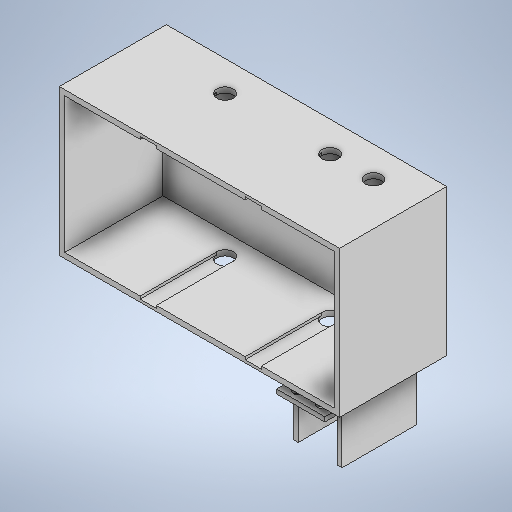
# Autodesk Inventor part: ClawHousing
Saved by Autodesk Inventor 2025.1 (Build 291241000, 241)
## iProperties
Created: 2024-12-07
Part Number: ClawHousing
Material: Generic
Document SubType Name: Modeling
Designer: ishaa
Density: 1 g/cm^3
Appearance: Default
Author: ishaa
Autodesk Inventor part; units mm, degrees
ref_plane "YZ Plane" through (0, 0, 0) normal (1, 0, 0) x (0, 1, 0)
ref_plane "XZ Plane" through (0, 0, 0) normal (0, 1, 0) x (-1, 0, 0)
ref_plane "XY Plane" through (0, 0, 0) normal (0, 0, 1) x (1, 0, 0)
sketch "Sketch1" plane through (0, 0, 0) normal (0, 0, 1) x (1, 0, 0)
  line L0 (78.5, 41) -> (-78.5, 41)
  line L1 (-78.5, 41) -> (-78.5, -41)
  line L2 (-78.5, -41) -> (78.5, -41)
  line L3 (78.5, -41) -> (78.5, 41)
  line L4 (78.5, 41) -> (-78.5, -41) construction
  line L5 (-78.5, 41) -> (78.5, -41) construction
  point P0 (0, 0)
  dimension "d0" = 157
  dimension "d1" = 82
  constraints: 12 end point, 2 midpoint, 2 parallel, 1 horizontal, 1 perpendicular
  measures "d0" distance of L2.end L1.end
  measures "d1" distance of L1.end L0.end
extrude "Extrusion1" add sketch "Sketch1" along normal blind 60
sketch "Sketch2" plane through (0, 0, 60) normal (0, 0, 1) x (1, 0, 0)
  line L0 (-78.5, 41) -> (-78.5, -41) projected
  line L1 (-78.5, -41) -> (78.5, -41) projected
  line L2 (78.5, -41) -> (78.5, 41) projected
  line L3 (78.5, 41) -> (-78.5, 41) projected
  line L4 (75.5, 38) -> (75.5, -38)
  line L5 (75.5, -38) -> (-75.5, -38)
  line L6 (-75.5, -38) -> (-75.5, 38)
  line L7 (-75.5, 38) -> (75.5, 38)
  point P0 (0, 0)
  dimension "d4" = 3
  constraints: 8 end point, 3 other
  measures "d4" distance between parallel lines of L2 L4
extrude "Extrusion2" cut sketch "Sketch2" against normal blind 55 contours L4 L5 L6 L7
sketch "Sketch3" plane through (-78.5, -41, 0) normal (0, -1, 0) x (1, 0, 0)
  circle A0 centre (133, 17) radius 4.55 construction
  line L0 (0, 0) -> (157, 0) construction
  line L1 (133, 0) -> (133, 85.8256) construction
  line L2 (157, 0) -> (157, 60) construction
  circle A1 centre (108.668, 17) radius 4.55
  line L3 (154, 60) -> (3, 60) construction
  line L4 (0, 0) -> (0, 60) construction
  circle A2 centre (49.832, 17) radius 4.55
  line L5 (157, 17) -> (0, 17) construction
  circle A3 centre (133, 17) radius 6.75
  point P0 (78.5, 0)
  point P1 (128.45, 17)
  point P2 (113.218, 17)
  dimension "d7" = 9.1
  dimension "d11" = 9.1
  dimension "d15" = 9.1
  dimension "d19" = 24.332
  constraints: 8 point on line, 4 end point, 2 centre point, 2 coincident, 2 horizontal alignment, 1 perpendicular, 1 vertical, 5 other
  measures "d15" diameter of A2
  measures "d19" distance of point (133, 17) point (108.668, 17)
extrude "Extrusion3" cut sketch "Sketch3" against normal blind 60
sketch "Sketch4" plane through (-78.5, 41, 0) normal (0, 1, 0) x (1, 0, 0)
  circle A0 centre (49.832, -17) radius 4.55
  line L0 (157, -60) -> (0, -60) construction
  line L1 (157, 0) -> (157, -60) construction
  line L2 (157, 0) -> (0, 0) construction
  line L3 (0, 0) -> (0, -60) construction
  circle A1 centre (133, -17) radius 6.75 construction
  circle A2 centre (133, -17) radius 4.55
  circle A3 centre (108.668, -17) radius 4.55
  dimension "d70" = 9.1
  dimension "d71" = 9.1
  dimension "d72" = 24.332
  constraints: 3 centre point, 2 coincident
  measures "d70" diameter of A2
  measures "d71" diameter of A3
  measures "d72" distance of A1.centre A3.centre
extrude "Extrusion4" cut sketch "Sketch4" against normal blind 55
sketch "Sketch5" plane through (0, 0, 0) normal (0, 0, -1) x (-1, 0, 0)
  line L0 (8, 13.8564) -> (16, 0) construction
  line L1 (16, 0) -> (8, -13.8564) construction
  line L2 (8, -13.8564) -> (-8, -13.8564) construction
  line L3 (-8, -13.8564) -> (-16, 0) construction
  line L4 (-16, 0) -> (-8, 13.8564) construction
  line L5 (-8, 13.8564) -> (8, 13.8564) construction
  circle A0 centre (-8, 13.8564) radius 1.675
  circle A1 centre (-16, 0) radius 1.675
  circle A2 centre (-8, -13.8564) radius 1.675
  circle A3 centre (8, -13.8564) radius 1.675
  circle A4 centre (16, 0) radius 1.675
  circle A5 centre (8, 13.8564) radius 1.675
  point P0 (0, 0)
  point P1 (0, 0)
  dimension "d31" = 32
  dimension "d32" = 3.35
  dimension "d35" = 360
  constraints: 12 end point, 6 centre point, 2 coincident, 26 other
  measures "d31" distance of L0.end L3.end
  measures "d32" diameter of A0
extrude "Extrusion5" cut sketch "Sketch5" against normal blind 55
chamfer "Chamfer1" distance 1 angle 45 6 edges at (-6.325, -13.8564, 0) (9.675, -13.8564, 0) (17.675, 0, 0) (9.675, 13.8564, 0) (-6.325, 13.8564, 0) (-14.325, 0, 0)
sketch "Sketch6" plane through (0, 0, 0) normal (0, 0, -1) x (-1, 0, 0)
  line L0 (0, -4.344) -> (-3.762, -2.172)
  line L1 (-3.762, -2.172) -> (-3.762, 2.172)
  line L2 (-3.762, 2.172) -> (0, 4.344)
  line L3 (0, 4.344) -> (3.762, 2.172)
  line L4 (3.762, 2.172) -> (3.762, -2.172)
  line L5 (3.762, -2.172) -> (0, -4.344)
  point P0 (0, 0)
  point P1 (0, 0)
  constraints: 12 end point, 1 coincident, 13 other
extrude "Extrusion6" cut sketch "Sketch6" against normal blind 55
fillet "Fillet1" radius 3.175 6 edges at (-1.881, 3.258, 0) (-3.762, 0, 0) (-1.881, -3.258, 0) (1.881, -3.258, 0) (3.762, 0, 0) (1.881, 3.258, 0)
sketch "Sketch7" plane through (-78.5, -41, 0) normal (0, -1, 0) x (1, 0, 0)
  line L0 (123, 47.211) -> (143, 47.211) construction
  line L1 (143, 47.211) -> (143, 7.211) construction
  line L2 (143, 7.211) -> (123, 7.211) construction
  line L3 (123, 7.211) -> (123, 47.211) construction
  line L4 (144, 6.211) -> (144, 48.211)
  line L5 (144, 48.211) -> (122, 48.211)
  line L6 (122, 48.211) -> (122, 6.211)
  line L7 (122, 6.211) -> (144, 6.211)
  line L8 (146.54, 3.671) -> (146.54, 50.751)
  line L9 (146.54, 50.751) -> (119.46, 50.751)
  line L10 (119.46, 50.751) -> (119.46, 3.671)
  line L11 (119.46, 3.671) -> (146.54, 3.671)
  point P0 (78.5, 0)
  point P1 (133, 17)
  dimension "d47" = 20
  dimension "d48" = 40
  dimension "d49" = 9.789
  dimension "d50" = 1
  dimension "d51" = 2.54
  constraints: 24 end point, 6 parallel, 3 perpendicular, 1 horizontal, 6 other
  measures "d47" distance of L1.end L2.end
  measures "d48" distance of L0.end L1.end
  measures "d49" distance from line of L2 point (133, 17)
  measures "d50" distance between parallel lines of L1 L4
  measures "d51" distance between parallel lines of L7 L11
extrude "Extrusion7" add sketch "Sketch7" along normal blind 8.6
sketch "Sketch8" plane through (-78.5, -49.6, 0) normal (0, -1, 0) x (1, 0, 0)
  line L0 (144, 48.211) -> (144, 6.211) construction
  line L1 (144, 27.211) -> (146.54, 27.211) construction
  line L2 (146.54, 3.671) -> (146.54, 50.751) construction
  line L3 (146.54, 48.211) -> (144, 48.211)
  line L4 (144, 48.211) -> (144, 6.211)
  line L5 (144, 6.211) -> (146.54, 6.211)
  line L6 (146.54, 6.211) -> (146.54, 48.211)
  line L7 (146.54, 48.211) -> (144, 6.211) construction
  line L8 (144, 48.211) -> (146.54, 6.211) construction
  line L9 (119.46, 3.671) -> (146.54, 3.671) construction
  line L10 (133, 3.671) -> (133, 50.751) construction
  line L11 (146.54, 50.751) -> (119.46, 50.751) construction
  line L12 (122, 48.211) -> (122, 6.211) construction
  line L13 (119.46, 3.671) -> (119.46, 50.751) construction
  line L14 (119.46, 48.211) -> (122, 48.211)
  line L15 (122, 48.211) -> (122, 6.211)
  line L16 (122, 6.211) -> (119.46, 6.211)
  line L17 (119.46, 6.211) -> (119.46, 48.211)
  point P0 (78.5, 0)
  point P1 (145.27, 27.211)
  constraints: 28 end point, 7 midpoint, 5 symmetric about line, 2 parallel, 1 horizontal, 1 perpendicular
extrude "Extrusion8" add sketch "Sketch8" along normal blind 27
sketch "Sketch9" plane through (40.96, -41, 50.751) normal (0, 0, 1) x (1, 0, 0)
  line L0 (27.08, 0) -> (27.08, -8.6) projected
  line L1 (0, 0) -> (0, -8.6) projected
  line L2 (27.08, -8.6) -> (0, -8.6)
  line L3 (0, -8.6) -> (0, -6.1)
  line L4 (0, -6.1) -> (27.08, -6.1)
  line L5 (27.08, -6.1) -> (27.08, -8.6)
  point P0 (-40.96, 41)
  point P1 (27.08, -6.1)
  dimension "d56" = 2.5
  constraints: 8 end point, 2 parallel, 1 horizontal, 1 perpendicular, 1 point on line
  measures "d56" distance of L2.end L3.end
extrude "Extrusion9" add sketch "Sketch9" along normal blind 7
sketch "Sketch10" plane through (68.04, -41, 3.671) normal (0, 0, -1) x (-1, 0, 0)
  line L0 (2.54, -8.6) -> (0, -8.6) projected
  line L1 (27.08, 0) -> (27.08, -8.6) projected
  line L2 (0, -8.6) -> (27.08, -8.6)
  line L3 (27.08, -8.6) -> (27.08, -6.1)
  line L4 (27.08, -6.1) -> (0, -6.1)
  line L5 (0, -6.1) -> (0, -8.6)
  point P0 (68.04, 41)
  point P1 (2.54, -8.6)
  dimension "d59" = 2.5
  constraints: 8 end point, 2 parallel, 1 horizontal, 1 perpendicular, 1 point on line
  measures "d59" distance of L3.end L2.end
extrude "Extrusion10" add sketch "Sketch10" along normal blind 7
sketch "Sketch11" plane through (-78.5, -49.6, 0) normal (0, -1, 0) x (1, 0, 0)
  circle A0 centre (139.6, 53.06) radius 2.25
  line L0 (122, 48.211) -> (144, 48.211) projected
  line L1 (146.54, 48.211) -> (146.54, 57.751) projected
  line L2 (133, 48.211) -> (133, 57.751) construction
  line L3 (119.46, 57.751) -> (146.54, 57.751) construction
  circle A1 centre (126.4, 53.06) radius 2.25
  line L4 (144, 6.211) -> (144, 48.211) construction
  line L5 (144, 48.211) -> (144, 6.211) construction
  line L6 (144, 27.211) -> (121.61, 27.211) construction
  circle A2 centre (139.6, 1.362) radius 2.25
  circle A3 centre (126.4, 1.362) radius 2.25
  line L7 (144, 48.211) -> (144, 57.751) construction
  point P0 (78.5, 0)
  dimension "d63" = 4.5
  dimension "d64" = 4.849
  dimension "d68" = 4.4
  constraints: 6 end point, 4 centre point, 3 midpoint, 3 symmetric about line, 1 horizontal, 1 perpendicular, 1 point on line, 3 other
  measures "d63" diameter of A0
  measures "d64" distance from line of L0 A0.centre
  measures "d68" distance from line of L7 A0.centre
extrude "Extrusion11" cut sketch "Sketch11" against normal blind 5
sketch "Sketch12" plane through (-75.5, -38, 60) normal (0, 1, 0) x (1, 0, 0)
  circle A0 centre (105.668, 43) radius 4.55 projected
  arc A1 (101.118, 43) -> (110.218, 43) centre (105.668, 43) ccw
  circle A2 centre (46.832, 43) radius 4.55 projected
  circle A3 centre (105.668, 43) radius 4.55 projected
  circle A4 centre (130, 43) radius 6.75 projected
  line L0 (151, 0) -> (0, 0) projected
  line L1 (151, 0) -> (151, 55) projected
  line L2 (151, 55) -> (0, 55) projected
  line L3 (0, 0) -> (0, 55) projected
  circle A5 centre (105.668, 43) radius 4.55 projected
  line L4 (110.218, 43) -> (110.218, 5.168)
  line L5 (110.218, 5.168) -> (110.218, 0)
  line L6 (101.118, 43) -> (101.118, 0)
  line L7 (0, 0) -> (151, 0) projected
  line L8 (105.668, 43) -> (46.832, 43) construction
  line L9 (151, 0) -> (0, 0) construction
  line L10 (76.25, 43) -> (76.25, 1.2107) construction
  circle A6 centre (46.832, 43) radius 4.55
  arc A7 (42.282, 43) -> (51.382, 43) centre (46.832, 43) ccw
  line L11 (42.282, 43) -> (42.282, 5.168)
  line L12 (42.282, 5.168) -> (42.282, 0)
  line L13 (51.382, 43) -> (51.382, 0)
  arc A8 (51.382, 43) -> (42.282, 43) centre (46.832, 43) ccw construction
  circle A9 centre (46.832, 43) radius 4.55 projected
  arc A10 (51.382, 43) -> (42.282, 43) centre (46.832, 43) ccw
  point P0 (75.5, 60)
  constraints: 16 end point, 12 point on circle, 7 symmetric about line, 5 centre point, 4 coincident, 2 perpendicular, 2 point on line, 2 vertical, 1 horizontal, 1 midpoint, 2 other
extrude "Extrusion12" cut sketch "Sketch12" against normal blind 1.5 contours L4 L5 L0 L6 A0 | L0 L12 L11 A2 L13
sketch "Sketch13" plane through (-75.5, 38, 60) normal (0, -1, 0) x (1, 0, 0)
  circle A0 centre (46.832, -43) radius 4.55 projected
  arc A1 (42.282, -43) -> (51.382, -43) centre (46.832, -43) ccw
  circle A2 centre (105.668, -43) radius 4.55 projected
  arc A3 (101.118, -43) -> (110.218, -43) centre (105.668, -43) ccw
  line L0 (42.282, -43) -> (42.282, 0)
  line L1 (0, 0) -> (151, 0) projected
  line L2 (51.382, -43) -> (51.382, 0)
  line L3 (110.218, -43) -> (110.218, 0)
  line L4 (101.118, -43) -> (101.118, 0)
  point P0 (75.5, -60)
  constraints: 8 end point, 8 point on circle, 3 point on line, 2 centre point, 2 coincident, 2 parallel, 2 tangent, 1 perpendicular, 1 vertical
extrude "Extrusion13" cut sketch "Sketch13" against normal blind 1.5 contours A0 L0 L1 L2 | A2 L4 L1 L3
body "Solid1"
